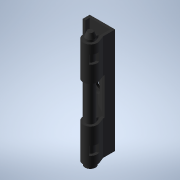
# Autodesk Inventor part: 1XXX_01_04(T,2)_P7
Saved by Autodesk Inventor 2021 (Build 250183000, 183)
## iProperties
Created: 2025-08-26
Part Number: 1XXX_01_04(T,2)_P7
Material: Generic
Catalog Web Link: www.cadenas.de
Description: AE 2.0 Scharnier-AE 2.0 Scharnier
Vendor: RITTAL
Document SubType Name: Modeling
Designer: psAdmin
Manufacturer: RITTAL
Mass: 4.76553 g
Surface Area: 56.6411 cm^2
Volume: 4.76553 cm^3
Density: 1 g/cm^3
Appearance: PSOLRGB-176-176-176
Category: PARTsolutions
Company: RITTAL
Title: 1XXX_01_04(T,2)_P7
Author: Cadenas PARTsolutions
Comments: AE 2.0 Scharnier
PSOL_IDENT_0: {$CADENAS_DATA/23d-libs/rittal/schaltschranksys/kompakt_schaltschr/parts_ae_2_0/scharnier_ae_2_0.prj
PSOL_IDENT_1: },203 {VTYP=3D},{NB=1XXX_01_04(T,2)_P7},{LINA=1XXX_01_04(T,2)_P7},{NN=AE 2.0 Scharnier},{DATE=28.04.
PSOL_IDENT_2: 2025 21:11:32},{GEOMDATE=11.04.2025 11:21:47},{VERSION=},{LINEID=410},{WBVAR=DETAIL,PIN},{WBNUMERIC=
PSOL_IDENT_3: DETAIL}  {NB=1XXX_01_04(T,2)_P7},{LINA=1XXX_01_04(T,2)_P7},{KT=DUMMY},{BEST=1XXX},{DETAIL=2},{PIN=T}
PSOL_IDENT_4: ,{BEZ1=Neues Kompaktgehäuse},{BEZ2=Stahlblech},{BEZ3=eintürig},{B=300},{H=300},{VERS=3},{W=294},{W1=
PSOL_IDENT_5: 225},{HH=294},{H1=175},{H2=240},{H4=59.5},{H5=0.000},{D=16.5},{ST=1.5},{R1=5.0},{GEW=-1.000000015047
PSOL_IDENT_6: 47e+30},{CNSECLASS51=27-18-01-02},{CNSECLASS70=27-18-01-01},{CNSECLASS80=27-18-01-01},{CNSETIM40=EC0
PSOL_IDENT_7: 00261}
NB: 1XXX_01_04(T,2)_P7
NN: AE 2.0 Scharnier
NT: AE 2.0 Scharnier
NBSYN: $BEST._01_04($PIN.,$DETAIL.)_P7
LINA: 1XXX_01_04(T,2)_P7
CATALOG: Rittal
BEST: 1XXX
DETAIL: niedrig
PIN: Top
BEZ1: Neues Kompaktgehäuse
BEZ2: Stahlblech
BEZ3: eintürig
B: 300
H: 300
VERS: 3
W: 294
W1: 225
HH: 294
H1: 175
H2: 240
H4: 59.5
H5: 0
D: 16.5
ST: 1.5
R1: 5
GEW: -1.00000001504747e+30
CNSECLASS70: 27-18-01-01
CNSECLASS80: 27-18-01-01
SUPPLIER: RITTAL
ARTICLENO: 1XXX_01_04(T,2)_P7
BOMINFO: 1XXX_01_04(T,2)_P7
CREATOR: CADENAS GmbH
Autodesk Inventor part; units mm, degrees
sketch "Sketch_12" plane through (0, 0, 0) normal (0, 1, 0) x (-1, 0, 0)
  line L0 (5.5, 3.4) -> (-1.2, 3.4)
  line L1 (-1.2, 3.4) -> (-6, 5.984)
  line L2 (-6, 5.984) -> (-6, 1.5)
  line L3 (-6, 1.5) -> (5.5, 1.5)
  line L4 (5.5, 1.5) -> (5.5, 3.4)
  constraints: 10 end point
extrude "Extrusion1" add sketch "Sketch_12" along normal mid plane 17.3
sketch "Sketch_16" plane through (0, 0, 0) normal (0, 0, 1) x (1, 0, 0)
  circle A0 centre (0, 0) radius 3.5
  constraints: 1 centre point
extrude "Extrusion2" cut sketch "Sketch_16" along normal blind 6
sketch "Sketch_1" plane through (0, 0, 0) normal (0, 1, 0) x (0, 0, 1)
  line L0 (0, 7.5) -> (0, -7)
  line L1 (0, -7) -> (4, -7)
  line L2 (4, -7) -> (4, -5.5)
  line L3 (4, -5.5) -> (1.5, -5.5)
  line L4 (1.5, -5.5) -> (1.5, 6)
  line L5 (1.5, 6) -> (7.1676, 6)
  line L6 (7.1676, 6) -> (10.6991, 7.3911)
  arc A0 (9.0682, 5.2618) -> (10.6991, 7.3911) centre (11.652, 4.972) ccw
  line L7 (9.0682, 5.2618) -> (7.5776, 5.429)
  arc A1 (7.5776, 5.429) -> (10.1493, 8.7867) centre (11.652, 4.972) ccw
  line L8 (10.1493, 8.7867) -> (6.8828, 7.5)
  line L9 (6.8828, 7.5) -> (0, 7.5)
  constraints: 20 end point, 4 point on circle, 2 centre point
extrude "Extrusion3" add sketch "Sketch_1" along normal mid plane 60
sketch "Sketch_8" plane through (0, 22.5, 0) normal (0, 1, 0) x (0, 0, 1)
  arc A0 (7.1855, 5.5204) -> (8.6409, 1.6278) centre (11.652, 4.972) ccw
  line L0 (8.6409, 1.6278) -> (9.9792, 3.1141)
  arc A1 (9.9792, 3.1141) -> (13.622, 6.5112) centre (11.652, 4.972) ccw
  line L1 (13.622, 6.5112) -> (15.198, 7.7425)
  arc A2 (15.198, 7.7425) -> (10.2614, 9.2518) centre (11.652, 4.972) ccw
  line L2 (10.2614, 9.2518) -> (10.8795, 7.3496)
  arc A3 (10.8795, 7.3496) -> (9.1706, 5.2767) centre (11.652, 4.972) ccw
  line L3 (9.1706, 5.2767) -> (7.1855, 5.5204)
  constraints: 8 end point, 8 point on circle, 4 centre point
extrude "Extrusion4" cut sketch "Sketch_8" along normal mid plane 5
sketch "Sketch_9" plane through (0, -22.5, 0) normal (0, 1, 0) x (0, 0, 1)
  arc A0 (7.1855, 5.5204) -> (8.6409, 1.6278) centre (11.652, 4.972) ccw
  line L0 (8.6409, 1.6278) -> (9.9792, 3.1141)
  arc A1 (9.9792, 3.1141) -> (13.622, 6.5112) centre (11.652, 4.972) ccw
  line L1 (13.622, 6.5112) -> (15.198, 7.7425)
  arc A2 (15.198, 7.7425) -> (10.2614, 9.2518) centre (11.652, 4.972) ccw
  line L2 (10.2614, 9.2518) -> (10.8795, 7.3496)
  arc A3 (10.8795, 7.3496) -> (9.1706, 5.2767) centre (11.652, 4.972) ccw
  line L3 (9.1706, 5.2767) -> (7.1855, 5.5204)
  constraints: 8 end point, 8 point on circle, 4 centre point
extrude "Extrusion5" cut sketch "Sketch_9" along normal mid plane 5
sketch "Sketch_5" plane through (0, 0, 0) normal (0, 1, 0) x (0, 0, 1)
  line L0 (1.5, 0) -> (0, 0)
  line L1 (0, 0) -> (0, 2.517)
  arc A0 (0, 2.517) -> (0.45, 2.067) centre (0.45, 2.517) ccw
  line L2 (0.45, 2.067) -> (1.5, 2.067)
  line L3 (1.5, 2.067) -> (1.5, 0)
  line L4 (1.5, 0) -> (0, 0)
  constraints: 10 end point, 2 point on circle, 1 centre point
revolve "Revolution1" cut sketch "Sketch_5" angle 360 about axis through (0, 0, 1.5) along (0, 0, 1)
thread "Thread1" size "M5x0.8" class "6H" standard "ISO Metric profile" full length
sketch "Sketch_6" plane through (7.5, 0, 0) normal (-1, 0, 0) x (0, 0, 1)
  line L0 (5.984, -10.5) -> (15.984, -10.5)
  line L1 (15.984, -10.5) -> (15.984, 10.5)
  line L2 (15.984, 10.5) -> (5.984, 10.5)
  line L3 (5.984, 10.5) -> (5.984, -10.5)
  constraints: 8 end point
extrude "Extrusion6" cut sketch "Sketch_6" along normal mid plane 14
sketch "Sketch_7" plane through (0, 0, 11.652) normal (0, 0, 1) x (1, 0, 0)
  line L0 (4.972, -32.2) -> (4.972, 33.8)
  line L1 (4.972, 33.8) -> (6.472, 33.8)
  line L2 (6.472, 33.8) -> (7.472, 31.05)
  line L3 (7.472, 31.05) -> (7.472, -26.7)
  line L4 (7.472, -26.7) -> (7.572, -26.7)
  line L5 (7.572, -26.7) -> (7.572, -27.7)
  line L6 (7.572, -27.7) -> (6.722, -27.7)
  line L7 (6.722, -27.7) -> (6.722, -30.7)
  line L8 (6.722, -30.7) -> (7.972, -30.7)
  line L9 (7.972, -30.7) -> (7.972, -32.2)
  line L10 (7.972, -32.2) -> (4.972, -32.2)
  line L11 (4.972, -32.2) -> (4.972, 33.8)
  constraints: 24 end point
revolve "Revolution2" add sketch "Sketch_7" angle 360 about axis through (4.972, -32.2, 11.652) along (0, -1, 0)
ref_plane "SC_XY" through (0, 0, 0) normal (0, 0, 1) x (-1, 0, 0)
ref_plane "SC_YZ" through (0, 0, 0) normal (-1, 0, 0) x (0, -1, 0)
ref_plane "SC_ZX" through (0, 0, 0) normal (0, -1, 0) x (0, 0, 1)
ref_plane "TUER1_XY" through (4.972, 0, 11.652) normal (0, -1, 0) x (0, 0, 1)
ref_plane "TUER1_YZ" through (4.972, 0, 11.652) normal (0, 0, 1) x (-1, 0, 0)
ref_plane "TUER1_ZX" through (4.972, 0, 11.652) normal (-1, 0, 0) x (0, -1, 0)
ref_plane "TUER2_XY" through (4.972, 0, 11.652) normal (0, 1, 0) x (0, 0, 1)
ref_plane "TUER2_YZ" through (4.972, 0, 11.652) normal (0, 0, 1) x (1, 0, 0)
ref_plane "TUER2_ZX" through (4.972, 0, 11.652) normal (1, 0, 0) x (0, 1, 0)
body "Solid1"
